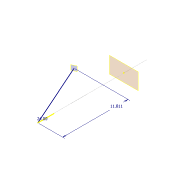
# Autodesk Inventor part: 00_Beampath_v0
Saved by Autodesk Inventor 2022 (Build 260153000, 153)
## iProperties
Created: 2022-04-09
Part Number: 00_Beampath_v0
Material: Generic
Document SubType Name: Modeling
Designer: Prakash Lab
Density: 1 g/cm^3
Appearance: Default
Author: Prakash Lab
Autodesk Inventor part; units mm, degrees
ref_plane "YZ Plane" through (0, 0, 0) normal (1, 0, 0) x (0, 1, 0)
ref_plane "XZ Plane" through (0, 0, 0) normal (0, 1, 0) x (-1, 0, 0)
ref_plane "XY Plane" through (0, 0, 0) normal (0, 0, 1) x (1, 0, 0)
ref_plane "Work Plane1" through (0, 0, 0) normal (0, 0, 1) x (1, 0, 0)
sketch "Sketch1" plane through (0, 0, 0) normal (0, 0, 1) x (1, 0, 0)
  circle A0 centre (0, 0) radius 0.5
  dimension "d0" = 1
  constraints: 1 centre point, 1 coincident
  measures "d0" diameter of A0
extrude "Extrusion1" add sketch "Sketch1" along normal blind 170 and the other way blind 105
sketch "Sketch2" plane through (0, 0, 170) normal (0, 0, 1) x (1, 0, 0)
  circle A0 centre (0, 0) radius 0.5 projected
  circle A1 centre (0, 0) radius 0.8208
  constraints: 1 centre point, 1 coincident
extrude "Extrusion2" add sketch "Sketch2" along normal blind 75 contours A0 | A1
sketch "Sketch3" plane through (0, 0, 245) normal (0, 0, 1) x (1, 0, 0)
  circle A0 centre (0, 0) radius 0.8208 projected
  circle A1 centre (0, 0) radius 0.5 projected
  circle A2 centre (0, 0) radius 0.5
  constraints: 1 centre point, 1 coincident
extrude "Extrusion3" add sketch "Sketch3" along normal blind 75 contours A1
sketch "Sketch4" plane through (0, 0, 320) normal (0, 0, 1) x (1, 0, 0)
  circle A0 centre (0, 0) radius 0.8208 projected
extrude "Extrusion4" add sketch "Sketch4" along normal blind 75
sketch "Sketch5" plane through (0, 0, 0) normal (0, 1, 0) x (-1, 0, 0)
  line L0 (-0.8208, 320) -> (-0.8208, 395) projected
  line L1 (-0.8208, 320) -> (-0.8208, 395) projected
  line L2 (0.8208, 320) -> (0.8208, 395) projected
  line L3 (0.8208, 395) -> (-0.8208, 395) projected
  line L4 (0, 395) -> (133.5686, 95)
  point P0 (0, 0)
  dimension "d11" = 24
  dimension "d12" = 300
  constraints: 2 end point, 1 midpoint
  measures "d11" angle of L0 L4
  measures "d12" vertical distance of L4.start L4.end
ref_plane "Work Plane2" through (-133.5686, 0, 95) normal (-0.4067366, 0, -0.9135455) x (0, -1, 0)
sketch "Sketch6" plane through (-133.5686, 0, 95) normal (-0.4067366, 0, -0.9135455) x (0, -1, 0)
  circle A0 centre (0, 0) radius 0.7121
  point P0 (0, -160.661)
  constraints: 1 centre point
extrude "Extrusion5" add sketch "Sketch6" against normal up to surface surface through (0, 0, 395) normal (0, 0, 1)
body "Solid1"
